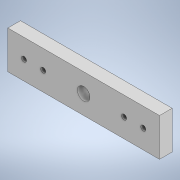
# Autodesk Inventor part: Solenoid Mounting Panel
Saved by Autodesk Inventor 2022 (Build 260153000, 153)
## iProperties
Created: 2022-01-19
Part Number: Solenoid Mounting Panel
Material: Generic
Document SubType Name: Modeling
Designer: gnzak
Density: 1 g/cm^3
Appearance: Default
Author: gnzak
Autodesk Inventor part; units mm, degrees
ref_plane "YZ Plane" through (0, 0, 0) normal (1, 0, 0) x (0, 1, 0)
ref_plane "XZ Plane" through (0, 0, 0) normal (0, 1, 0) x (-1, 0, 0)
ref_plane "XY Plane" through (0, 0, 0) normal (0, 0, 1) x (1, 0, 0)
sketch "Sketch2" plane through (0, 0, 0) normal (0, 0, 1) x (1, 0, 0)
  line L0 (-38.1, 9.525) -> (38.1, 9.525)
  line L1 (38.1, 9.525) -> (38.1, -9.525)
  line L2 (38.1, -9.525) -> (-38.1, -9.525)
  line L3 (-38.1, -9.525) -> (-38.1, 9.525)
  point P0 (0, 0)
  dimension "d0" = 76.2
  dimension "d1" = 19.05
  dimension "d2" = 38.1
  dimension "d3" = 9.525
  constraints: 8 end point, 2 parallel, 1 horizontal, 1 perpendicular
  measures "d0" distance of L0.start L0.end
  measures "d1" distance of L2.end L0.start
  measures "d2" distance from line of point (0, 0) L3
  measures "d3" distance from line of point (0, 0) L0
extrude "Extrusion1" add sketch "Sketch2" along normal blind 6.35
sketch "Sketch3" plane through (0, 0, 6.35) normal (0, 0, 1) x (1, 0, 0)
  circle A0 centre (0, 0) radius 3.175
  circle A1 centre (-20.32, 0) radius 1.27
  circle A2 centre (20.32, 0) radius 1.27
  circle A3 centre (0, 0) radius 10.16
  circle A4 centre (-29.972, 0) radius 1.27
  circle A5 centre (29.972, 0) radius 1.27
  dimension "d6" = 6.35
  dimension "d7" = 2.54
  dimension "d10" = 2.54
  dimension "d12" = 20.32
  dimension "d13" = 20.32
  dimension "d15" = 0
  dimension "d16" = 20.32
  dimension "d18" = 0
  dimension "d22" = 2.54
  dimension "d24" = 0
  dimension "d26" = 9.652
  dimension "d27" = 2.54
  dimension "d28" = 9.652
  dimension "d29" = 0
  constraints: 6 centre point, 2 coincident
  measures "d6" diameter of A0
  measures "d7" diameter of A1
  measures "d10" diameter of A2
  measures "d12" distance of point (0, 0) A1.centre
  measures "d13" diameter of A3
  measures "d15" vertical distance of point (0, 0) A1.centre
  measures "d16" distance of point (0, 0) A2.centre
  measures "d18" vertical distance of point (0, 0) A2.centre
  measures "d22" diameter of A4
  measures "d24" vertical distance of point (0, 0) A4.centre
  measures "d26" distance of A1.centre A4.centre
  measures "d27" diameter of A5
  measures "d28" distance of A2.centre A5.centre
  measures "d29" vertical distance of point (0, 0) A5.centre
extrude "Extrusion4" cut sketch "Sketch3" against normal blind 25.4 contours A0 | A1 | A2 | A4 | A5
equation "\"d2\" = 0.5 * d0"
equation "\"d3\" = 0.5 * d1"
equation "\"d16\" = d12"
body "Solid1"
